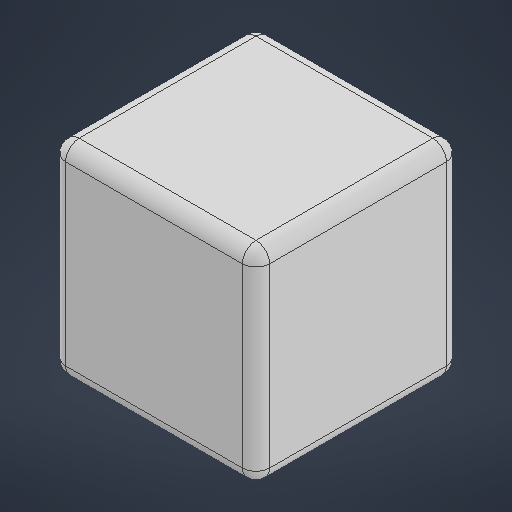
# Autodesk Inventor part: initial-rubbish-group2
Saved by Autodesk Inventor 2026.1 (Build 301233000, 233)
## iProperties
Created: 2026-02-25
Part Number: initial-rubbish-group2
Material: Generic
Document SubType Name: Modeling
Designer: ts2104
Density: 1 g/cm^3
Appearance: Default
Author: ts2104
Autodesk Inventor part; units mm, degrees
ref_plane "YZ Plane" through (0, 0, 0) normal (1, 0, 0) x (0, 1, 0)
ref_plane "XZ Plane" through (0, 0, 0) normal (0, 1, 0) x (-1, 0, 0)
ref_plane "XY Plane" through (0, 0, 0) normal (0, 0, 1) x (1, 0, 0)
sketch "Sketch1" plane through (0, 0, 0) normal (0, 0, 1) x (1, 0, 0)
  line L0 (-15, 15) -> (15, 15)
  line L1 (15, 15) -> (15, -15)
  line L2 (15, -15) -> (-15, -15)
  line L3 (-15, -15) -> (-15, 15)
  line L4 (-15, 15) -> (15, -15) construction
  line L5 (15, 15) -> (-15, -15) construction
  point P0 (0, 0)
  dimension "d0" = 30
  constraints: 12 end point, 2 midpoint, 2 parallel, 2 perpendicular, 1 horizontal
  measures "d0" distance of L2.end L0.start
extrude "Extrusion1" add sketch "Sketch1" along normal blind 30
fillet "Fillet1" radius 2 12 edges at (0, -15, 30) (0, -15, 0) (15, -15, 15) (15, 0, 30) (15, 0, 0) (15, 15, 15) (0, 15, 30) (0, 15, 0) (-15, 15, 15) (-15, 0, 30) (-15, -15, 15) (-15, 0, 0)
equation "\"d1\" = d0"
body "Solid1"
